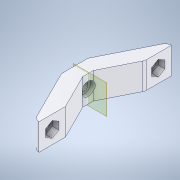
# Autodesk Inventor part: Bottom_Foot_Standoff
Saved by Autodesk Inventor 2021 (Build 250183000, 183)
## iProperties
Created: 2021-10-10
Part Number: Bottom_Foot_Standoff
Material: PET Plastic
Document SubType Name: Modeling
Designer: Jorian Brusind
Density: 1.541 g/cm^3
Appearance: PTFE
Mass: 35.6364 g
Surface Area: 72.3109 cm^2
Volume: 23.1255 cm^3
Author: Jorian Brusind
Autodesk Inventor part; units mm, degrees
ref_plane "YZ Plane" through (0, 0, 0) normal (1, 0, 0) x (0, 1, 0)
ref_plane "XZ Plane" through (0, 0, 0) normal (0, 1, 0) x (-1, 0, 0)
ref_plane "XY Plane" through (0, 0, 0) normal (0, 0, 1) x (1, 0, 0)
sketch "Sketch1" plane through (0, 0, 0) normal (0, 1, 0) x (-1, 0, 0)
  line L0 (0, 0) -> (-20, 0)
  line L1 (-20, 0) -> (-20, -40)
  line L2 (-20, -40) -> (0, 0)
  line L3 (-21.5, -50) -> (-18.5, -50)
  line L4 (-18.5, -50) -> (-18.5, -30)
  line L5 (-18.5, -30) -> (-21.5, -30)
  line L6 (-21.5, -30) -> (-21.5, -50)
  line L7 (-21.5, -50) -> (-18.5, -30) construction
  line L8 (-18.5, -50) -> (-21.5, -30) construction
  line L9 (1.5, 10) -> (-1.5, 10)
  line L10 (-1.5, 10) -> (-1.5, -10)
  line L11 (-1.5, -10) -> (1.5, -10)
  line L12 (1.5, -10) -> (1.5, 10)
  line L13 (1.5, 10) -> (-1.5, -10) construction
  line L14 (-1.5, 10) -> (1.5, -10) construction
  line L15 (-1.5, 10) -> (-21.5, -30)
  line L16 (1.5, -10) -> (-18.5, -50)
  line L17 (1.5, -10) -> (1.5, 10)
  line L18 (1.5, -10) -> (1.5, 10)
  line L19 (1.5, 10) -> (-8.5, 10)
  line L20 (-8.5, 10) -> (-8.5, -10)
  line L21 (-8.5, -10) -> (1.5, -10)
  line L22 (1.5, -10) -> (1.5, 10)
  line L23 (0, 0) -> (10, 0)
  line L24 (0, 0) -> (10, 0) construction
  line L25 (-20, 40) -> (0, 0)
  line L26 (-21.5, 50) -> (-18.5, 50)
  line L27 (-18.5, 50) -> (-18.5, 30)
  line L28 (-18.5, 30) -> (-21.5, 30)
  line L29 (-21.5, 30) -> (-21.5, 50)
  line L30 (-1.5, -10) -> (-1.5, 10)
  line L31 (-1.5, 10) -> (1.5, 10)
  line L32 (-1.5, -10) -> (-21.5, 30)
  line L33 (1.5, 10) -> (-18.5, 50)
  line L34 (1.5, 10) -> (1.5, -10)
  point P0 (-7.3579, -1.7157)
  point P1 (-11.5, -10)
  point P2 (-11.5, -10)
  point P3 (-8.5, -4)
  point P4 (-8.5, 4)
  dimension "d0" = 20
  dimension "d1" = 40
  dimension "d2" = 3
  dimension "d3" = 20
  dimension "d4" = 3
  dimension "d5" = 20
  dimension "d31" = 10
  dimension "d32" = 20
  dimension "d42" = 10
  dimension "d43" = 0
  constraints: 70 end point, 10 symmetric about line, 6 parallel, 5 horizontal, 5 midpoint, 4 perpendicular, 2 collinear, 1 point on line
  measures "d0" distance of L0.start L0.end
  measures "d1" distance of L0.end L1.end
  measures "d2" distance of L5.end L4.end
  measures "d3" distance of L4.end L3.end
  measures "d4" distance of L11.end L10.end
  measures "d5" distance of L10.end L9.end
  measures "d31" distance of L21.end L20.end
  measures "d32" distance of L20.end L19.end
  measures "d42" distance of L0.start L23.end
  measures "d43" distance between parallel lines of L24 L23
extrude "Extrusion1" add sketch "Sketch1" along normal blind 20 contours L2 L10 L0 | L23 L12 L11 L10 L2 | L25 L10 L9 L12 L23 | L0 L10 L25 | L10 L2 L32 L0 | L0 L15 L25 L10 | L10 L32 L2 | L25 L15 L10 | L15 L20 L0 | L32 L20 L19 L25 L15 | L32 L2 L21 L20 L15 | L0 L20 L32 | L32 L21 L2 | L11 L16 L4 L2 L21 | L9 L19 L25 L27 L33 | L15 L25 L19 | L20 L21 L2 L4 L5 L1 L15 | L32 L28 L27 L25 L19 L20 | L3 L6 L5 L1 L2 L4 | L27 L28 L29 L26 | L1 L5 L15 | L2 L1 L5 L4
sketch "Sketch2" plane through (-1.5, 0, -10) normal (-1, 0, 0) x (0, 0, 1)
  circle A0 centre (10, 10) radius 3
  line L0 (0, 0) -> (20, 0) projected
  line L1 (20, 0) -> (20, 20) projected
  point P0 (10, 0)
  dimension "d8" = 6
  dimension "d9" = 10
  dimension "d44" = 10
  constraints: 1 centre point
  measures "d8" diameter of A0
  measures "d9" distance from line of L0 A0.centre
  measures "d44" distance from line of L1 A0.centre
sketch "Sketch3" plane through (21.5, 0, -30) normal (1, 0, 0) x (0, 0, -1)
  circle A0 centre (10, 10) radius 3.25
  line L0 (0, 20) -> (20, 20) projected
  line L1 (20, 0) -> (20, 20) projected
  point P0 (-30, 0)
  dimension "d11" = 6.5
  dimension "d12" = 10
  dimension "d13" = 10
  constraints: 1 centre point
  measures "d11" diameter of A0
  measures "d12" distance from line of L0 A0.centre
  measures "d13" distance from line of L1 A0.centre
extrude "Extrusion2" cut sketch "Sketch2" against normal through all
extrude "Extrusion3" cut sketch "Sketch3" against normal through all
sketch "Sketch4" plane through (21.5, 0, -30) normal (1, 0, 0) x (0, 0, -1)
  circle A0 centre (10, 10) radius 3.25 projected
  line L0 (10, 15.7735) -> (15, 12.8868)
  line L1 (15, 12.8868) -> (15, 7.1132)
  line L2 (15, 7.1132) -> (10, 4.2265)
  line L3 (10, 4.2265) -> (5, 7.1132)
  line L4 (5, 7.1132) -> (5, 12.8868)
  line L5 (5, 12.8868) -> (10, 15.7735)
  line L6 (20, 0) -> (20, 20) projected
  point P0 (-30, 0)
  point P1 (10, 10)
  dimension "d19" = 10
  constraints: 12 end point, 1 coincident, 1 parallel, 13 other
  measures "d19" distance between parallel lines of L1 L4
extrude "Extrusion4" cut sketch "Sketch4" against normal blind 5
fillet "Fillet2" radius 5 1 edges at (21.5, 10, -30)
mirror "Mirror1" about plane through (0, 0, 0) normal (0, 0, 1) of "Extrusion4", "Extrusion3"
sketch "Sketch7" plane through (8.5, 0, 4) normal (1, 0, 0) x (0, 0, -1)
  circle A0 centre (4, 10) radius 3 projected
  circle A1 centre (4, 10) radius 5
  point P0 (4, 0)
  dimension "d52" = 10
  constraints: 1 centre point, 1 coincident
  measures "d52" diameter of A1
extrude "Extrusion6" cut sketch "Sketch7" along normal mid plane 6 contours A0 | A1
fillet "Fillet8" radius 5 2 edges at (-1.5, 10, 10) (-1.5, 10, -10)
fillet "Fillet9" radius 5 2 edges at (18.5, 10, 50) (18.5, 10, -50)
ref_plane "Work Plane1" through (0, 0, 0) normal (0, 0, 1) x (1, 0, 0)
body "Solid1"
